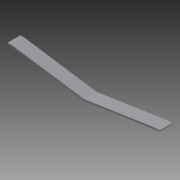
# Autodesk Inventor part: plough
Saved by Autodesk Inventor 2013 (Build 170138000, 138)
## iProperties
Created: 2013-02-04
Part Number: plough
Material: Generic
Document SubType Name: Modeling
Designer: Arpan
Density: 1 g/cm^3
Author: Arpan
Autodesk Inventor part; units mm, degrees
ref_plane "YZ Plane" through (0, 0, 0) normal (1, 0, 0) x (0, 1, 0)
ref_plane "XZ Plane" through (0, 0, 0) normal (0, 1, 0) x (-1, 0, 0)
ref_plane "XY Plane" through (0, 0, 0) normal (0, 0, 1) x (1, 0, 0)
sketch "Sketch1" plane through (0, 0, 0) normal (0, 0, 1) x (1, 0, 0)
  line L0 (0, 0) -> (0, 22.86)
  line L1 (-304.8, 0) -> (-304.8, 22.86)
  line L2 (-304.8, 22.86) -> (-152.4, 0)
  line L3 (-152.4, 0) -> (0, 22.86)
  line L4 (-304.8, 19.6495) -> (-173.8035, 0)
  line L5 (-130.9965, 0) -> (0, 19.6495)
  line L6 (-173.8035, 0) -> (-152.4, -3.2105)
  line L7 (-130.9965, 0) -> (-152.4, -3.2105)
  line L8 (-304.8, 0) -> (-173.8035, 0)
  line L9 (-130.9965, 0) -> (0, 0)
  line L10 (-152.4, -3.2105) -> (-165.1, -3.2105)
  line L11 (-165.1, -3.2105) -> (-165.1, -1.3055)
  dimension "d0" = 22.86
  dimension "d2" = 304.8
  dimension "d4" = 3.175
  dimension "d5" = 3.175
  dimension "d8" = 12.7
  constraints: 24 end point, 3 collinear, 3 parallel, 3 point on line, 2 perpendicular, 1 equal length, 1 vertical
  measures "d0" distance of L0.start L0.end
  measures "d2" distance of L0.start L1.start
  measures "d4" distance between parallel lines of L2 L4
  measures "d5" distance between parallel lines of L3 L5
  measures "d8" distance of L6.end L10.end
extrude "Extrusion1" add sketch "Sketch1" along normal blind 25.4 contours L5 L7 L6 L4 L1 L2 L3 L0
sketch "Sketch2" plane through (0, 0, 25.4) normal (0, 0, 1) x (1, 0, 0)
  line L0 (0, 19.6495) -> (0, 22.86) projected
  line L1 (0, 22.86) -> (-152.4, 0) projected
  line L2 (-152.4, 0) -> (-304.8, 22.86) projected
  line L3 (-304.8, 22.86) -> (-304.8, 19.6495) projected
  line L4 (-304.8, 22.86) -> (-304.8, 21.5646)
  line L5 (-304.8, 21.5646) -> (-296.164, 21.5646)
  line L6 (0, 22.86) -> (0, 21.5646)
  line L7 (0, 21.5646) -> (-10.7017, 21.2547)
  point P0 (0, 0)
  dimension "d9" = 1.2954
  dimension "d10" = 1.2954
  constraints: 8 end point, 4 point on line, 1 perpendicular
  measures "d9" distance of L2.end L4.end
  measures "d10" distance of L0.end L6.end
extrude "Extrusion2" cut sketch "Sketch2" against normal blind 50.8
body "Solid1"
